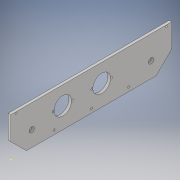
# Autodesk Inventor part: DriveTrainPlate
Saved by Autodesk Inventor 2017 (Build 210142000, 142)
## iProperties
Created: 2016-09-21
Part Number: DriveTrainPlate
Material: Generic
Document SubType Name: Modeling
Designer: RoboticsUser
Density: 1 g/cm^3
Appearance: Default
Author: RoboticsUser
Autodesk Inventor part; units mm, degrees
ref_plane "YZ Plane" through (0, 0, 0) normal (1, 0, 0) x (0, 1, 0)
ref_plane "XZ Plane" through (0, 0, 0) normal (0, 1, 0) x (-1, 0, 0)
ref_plane "XY Plane" through (0, 0, 0) normal (0, 0, 1) x (1, 0, 0)
sketch "Sketch1" plane through (0, 0, 0) normal (1, 0, 0) x (0, 1, 0)
  line L0 (444.5, 0) -> (444.5, -2.1042)
  line L1 (0, -2.1042) -> (0, 0)
  line L2 (0, -74.1174) -> (0, -66.8433)
  line L3 (0, 0) -> (95.25, 0)
  line L4 (95.25, 0) -> (95.25, -393.7)
  line L5 (95.25, -393.7) -> (0, -393.7)
  line L6 (0, -393.7) -> (0, 0)
  point P0 (38.1, -50.8)
  point P1 (38.1, -342.9)
  dimension "d2" = 95.25
  dimension "d3" = 393.7
  dimension "d4" = 50.8
  dimension "d5" = 38.1
  dimension "d6" = 50.8
  dimension "d7" = 38.1
  constraints: 14 end point, 3 parallel, 1 horizontal, 1 perpendicular, 1 point on line
  measures "d2" distance of L4.end L5.end
  measures "d3" distance of L3.end L4.end
  measures "d4" distance from line of L3 point (38.1, -50.8)
  measures "d5" distance from line of L6 point (38.1, -50.8)
  measures "d6" distance from line of L5 point (38.1, -342.9)
  measures "d7" distance from line of L6 point (38.1, -342.9)
extrude "Extrusion1" add sketch "Sketch1" along normal blind 6.35
sketch "Sketch3" plane through (6.35, 0, 0) normal (1, 0, 0) x (0, 0, -1)
  point P0 (0, 0)
sketch "Sketch4" plane through (6.35, 0, 0) normal (1, 0, 0) x (0, 0, -1)
  point P0 (0, 0)
chamfer "Chamfer1" distance 38.1 angle 45 1 edges at (3.175, 0, 0)
chamfer "Chamfer2" distance 38.1 angle 45 1 edges at (3.175, 0, -393.7)
sketch "Sketch5" plane through (0, 0, 0) normal (-1, 0, 0) x (0, 0, 1)
  line L0 (0, 95.25) -> (-393.7, 95.25) projected
  line L1 (-355.6, 0) -> (-393.7, 38.1) projected
  line L2 (-355.6, 0) -> (-38.1, 0) projected
  line L3 (0, 38.1) -> (-38.1, 0) projected
  line L4 (0, 38.1) -> (0, 95.25) projected
  line L5 (0, 95.25) -> (-393.7, 95.25) projected
  line L6 (-393.7, 95.25) -> (-393.7, 38.1) projected
  point P0 (0, 0)
  point P1 (-342.9, 38.1)
  point P2 (-50.8, 38.1)
  dimension "d16" = 50.8
  dimension "d17" = 38.1
  dimension "d18" = 38.1
  dimension "d19" = 50.8
  measures "d16" distance from line of L6 point (-342.9, 38.1)
  measures "d17" distance from line of point (-342.9, 38.1) L2
  measures "d18" distance from line of L2 point (-50.8, 38.1)
  measures "d19" distance from line of L4 point (-50.8, 38.1)
hole "Hole1" at (0, 38.1, -342.9) at (0, 38.1, -50.8) direction (1, 0, 0) diameter 12.7254 end through all
sketch "Sketch6" plane through (0, 0, 0) normal (-1, 0, 0) x (0, 0, 1)
  line L0 (-393.7, 95.25) -> (-393.7, 38.1) projected
  line L1 (-38.1, 0) -> (-355.6, 0) projected
  line L2 (0, 38.1) -> (0, 95.25) projected
  point P0 (0, 0)
  point P1 (-222.25, 50.8)
  point P2 (-127, 50.8)
  point P3 (-102.997, 50.8)
  point P4 (-151.003, 50.8)
  point P5 (-198.247, 50.8)
  point P6 (-246.253, 50.8)
  dimension "d27" = 171.45
  dimension "d28" = 50.8
  dimension "d29" = 127
  dimension "d30" = 50.8
  dimension "d31" = 24.003
  dimension "d32" = 24.003
  dimension "d33" = 24.003
  dimension "d34" = 24.003
  measures "d27" distance from line of L0 point (-222.25, 50.8)
  measures "d28" distance from line of L1 point (-222.25, 50.8)
  measures "d29" distance from line of L2 point (-127, 50.8)
  measures "d30" distance from line of L1 point (-127, 50.8)
  measures "d31" distance of point (-127, 50.8) point (-102.997, 50.8)
  measures "d32" distance of point (-127, 50.8) point (-151.003, 50.8)
  measures "d33" distance of point (-222.25, 50.8) point (-198.247, 50.8)
  measures "d34" distance of point (-246.253, 50.8) point (-222.25, 50.8)
hole "Hole2" at (0, 50.8, -246.253) at (0, 50.8, -222.25) at (0, 50.8, -198.247) at (0, 50.8, -102.997) at (0, 50.8, -127) at (0, 50.8, -151.003) direction (1, 0, 0) diameter 4.7752 end through all
sketch "Sketch7" plane through (0, 0, 0) normal (-1, 0, 0) x (0, 0, 1)
  line L0 (-38.1, 0) -> (-355.6, 0) projected
  line L1 (-393.7, 95.25) -> (-393.7, 38.1) projected
  line L2 (0, 38.1) -> (0, 95.25) projected
  line L3 (0, 95.25) -> (-393.7, 95.25) projected
  point P0 (0, 0)
  point P1 (-298.45, 10.0076)
  point P2 (-95.25, 10.0076)
  point P3 (-12.7, 91.5924)
  point P4 (-381, 91.5924)
  dimension "d42" = 10.0076
  dimension "d43" = 95.25
  dimension "d44" = 95.25
  dimension "d45" = 3.6576
  dimension "d46" = 12.7
  dimension "d47" = 12.7
  measures "d42" distance from line of L0 point (-298.45, 10.008)
  measures "d43" distance from line of L1 point (-298.45, 10.008)
  measures "d44" distance from line of L2 point (-95.25, 10.008)
  measures "d45" distance from line of L3 point (-12.7, 91.592)
  measures "d46" distance from line of point (-12.7, 91.592) L2
  measures "d47" distance from line of L1 point (-381, 91.592)
hole "Hole3" at (0, 91.5924, -381) at (0, 91.5924, -12.7) direction (1, 0, 0) diameter 4.7752 end through all
sketch "Sketch8" plane through (0, 0, 0) normal (-1, 0, 0) x (0, 0, 1)
  line L0 (0, 38.1) -> (0, 95.25) projected
  line L1 (0, 95.25) -> (-393.7, 95.25) projected
  line L2 (-355.6, 0) -> (-38.1, 0) projected
  point P0 (0, 0)
  point P1 (-196.85, 91.5924)
  point P2 (-196.85, 10.0076)
  dimension "d55" = 196.85
  dimension "d56" = 3.6576
  dimension "d57" = 10.0076
  measures "d55" distance from line of L0 point (-196.85, 91.592)
  measures "d56" distance from line of L1 point (-196.85, 91.592)
  measures "d57" distance from line of L2 point (-196.85, 10.008)
sketch "Sketch9" plane through (0, 0, 0) normal (-1, 0, 0) x (0, 0, 1)
  line L0 (-355.6, 0) -> (-38.1, 0) projected
  line L1 (-393.7, 95.25) -> (-393.7, 38.1) projected
  line L2 (0, 38.1) -> (0, 95.25) projected
  point P0 (0, 0)
  point P1 (-287.8836, 10.0076)
  point P2 (-105.8164, 10.0076)
  dimension "d58" = 10.0076
  dimension "d59" = 105.8164
  dimension "d60" = 105.8164
  measures "d58" distance from line of L0 point (-287.884, 10.008)
  measures "d59" distance from line of L1 point (-287.884, 10.008)
  measures "d60" distance from line of L2 point (-105.816, 10.008)
hole "Hole4" at (0, 10.0076, -196.85) direction (1, 0, 0) diameter 4.7752 end through all
hole "Hole5" at (0, 10.0076, -105.8164) at (0, 10.0076, -287.8836) direction (1, 0, 0) diameter 4.7752 end through all
sketch "Sketch10" plane through (0, 0, 0) normal (-1, 0, 0) x (0, 0, 1)
  circle A0 centre (-222.25, 50.8) radius 2.3876 projected
  circle A1 centre (-127, 50.8) radius 2.3876 projected
  point P0 (0, 0)
  point P1 (-127, 48.4124)
  constraints: 1 coincident, 1 vertical alignment, 1 other
hole "Hole6" at (0, 50.8, -222.25) at (0, 50.8, -127) direction (1, 0, 0) diameter 43.18 end through all
body "Solid1"
